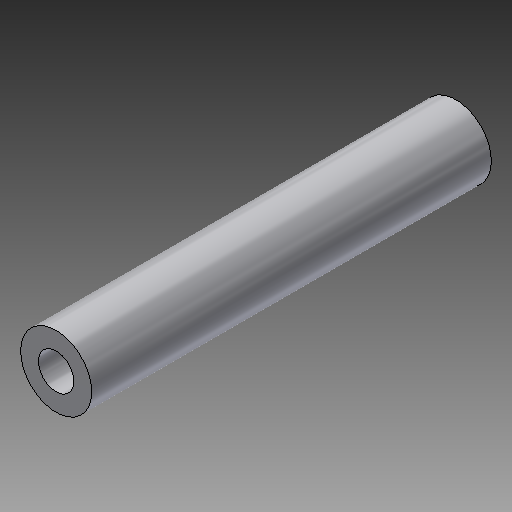
# Autodesk Inventor part: スペーサ　m4-l45
Saved by Autodesk Inventor 2019 (Build 230136000, 136)
## iProperties
Created: 2017-03-06
Part Number: スペーサ　m4-l45
Material: アルミニウム 2014-T4
Document SubType Name: Modeling
Designer: 大空
Density: 2.8 g/cm^3
Appearance: サテン
Mass: 5.74229 g
Surface Area: 14.3675 cm^2
Volume: 2.05082 cm^3
Author: 大空
Autodesk Inventor part; units mm, degrees
ref_plane "YZ Plane" through (0, 0, 0) normal (1, 0, 0) x (0, 1, 0)
ref_plane "XZ Plane" through (0, 0, 0) normal (0, 1, 0) x (-1, 0, 0)
ref_plane "XY Plane" through (0, 0, 0) normal (0, 0, 1) x (1, 0, 0)
sketch "スケッチ1" plane through (0, 0, 0) normal (0, 0, 1) x (1, 0, 0)
  circle A0 centre (0, 0) radius 4
  dimension "d0" = 8
  constraints: 1 centre point, 1 coincident
  measures "d0" diameter of A0
extrude "押し出し1" add sketch "スケッチ1" along normal blind 45
hole "穴1" at (0, 0, 0) direction (0, 0, 1) diameter 4 depth 8 tip angle 118
sketch "スケッチ2" plane through (0, 0, 45) normal (0, 0, 1) x (1, 0, 0)
  point P0 (0, 0)
  point P1 (0, 0)
  constraints: 1 coincident
hole "穴2" at (0, 0, 45) direction (0, 0, -1) diameter 4 depth 8 tip angle 118
